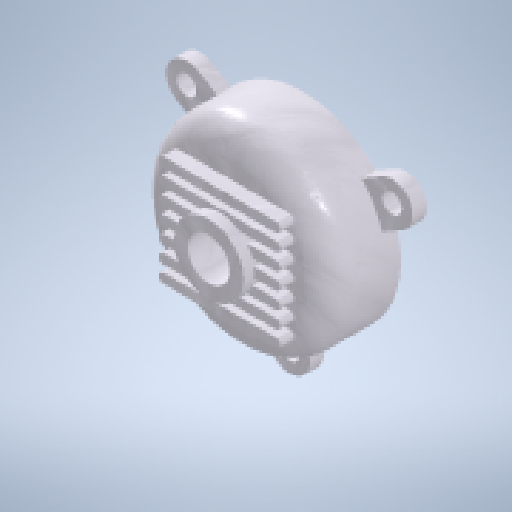
# Autodesk Inventor part: Disco do Motor Industrial
Saved by Autodesk Inventor 2023.2 (Build 272271000, 271)
## iProperties
Created: 2022-07-19
Part Number: Disco do Motor Industrial
Material: Aluminum 6061, Welded
Document SubType Name: Modeling
Designer: coqui
Density: 2.7 g/cm^3
Appearance: Weld - Aluminum
Mass: 46.1489 g
Surface Area: 212.112 cm^2
Volume: 17.0922 cm^3
Author: coqui
Autodesk Inventor part; units mm, degrees
ref_plane "YZ Plane" through (0, 0, 0) normal (1, 0, 0) x (0, 1, 0)
ref_plane "XZ Plane" through (0, 0, 0) normal (0, 1, 0) x (-1, 0, 0)
ref_plane "XY Plane" through (0, 0, 0) normal (0, 0, 1) x (1, 0, 0)
sketch "Sketch1" plane through (0, 0, 0) normal (0, 0, 1) x (1, 0, 0)
  circle A0 centre (0, 0) radius 35
  dimension "d0" = 70
  constraints: 1 centre point, 1 coincident
  measures "d0" diameter of A0
extrude "Extrusion1" add sketch "Sketch1" along normal blind 25
fillet "Fillet1" radius 10 1 edges at (-35, 0, 25)
shell "Shell1" thickness 1 removed faces 1 at (-1.9985, 11.019, 0)
sketch "Sketch2" plane through (0, 0, 0) normal (0, 0, -1) x (-1, 0, 0)
  arc A0 (-7.5, -42.5) -> (7.5, -42.5) centre (0, -42.5) ccw
  circle A1 centre (0, -42.5) radius 3.5
  line L0 (7.5, -42.5) -> (7.5, -33.6234)
  line L1 (-7.5, -42.5) -> (-7.5, -33.7627)
  arc A2 (-7.5, -33.7627) -> (7.5, -33.7627) centre (0, -11.6498) ccw
  point P0 (0, 0)
  dimension "d5" = 15
  dimension "d6" = 7
  dimension "d7" = 42.5
  constraints: 4 end point, 4 point on circle, 3 centre point, 1 coincident, 1 parallel, 1 point on line, 1 tangent, 1 vertical
  measures "d5" diameter of A0
  measures "d6" diameter of A1
  measures "d7" distance of A0.centre point (0, 0)
extrude "Extrusion2" add sketch "Sketch2" against normal blind 5
pattern_circular "Circular Pattern1" count 3 over 360 about axis through (0, 0, 15) along (0, 0, 1) of "Extrusion2"
sketch "Sketch3" plane through (0, 0, 25) normal (0, 0, 1) x (1, 0, 0)
  line L0 (20, 18) -> (-20, 18) construction
  line L1 (20, 19.75) -> (-20, 19.75)
  line L2 (-20, 16.25) -> (20, 16.25)
  arc A0 (20, 16.25) -> (20, 19.75) centre (20, 18) ccw
  arc A1 (-20, 19.75) -> (-20, 16.25) centre (-20, 18) ccw
  line L3 (0, 42.0299) -> (0, -57.656) construction
  line L4 (20, 12) -> (-20, 12) construction
  line L5 (20, 13.75) -> (-20, 13.75)
  line L6 (-20, 10.25) -> (20, 10.25)
  arc A2 (20, 10.25) -> (20, 13.75) centre (20, 12) ccw
  arc A3 (-20, 13.75) -> (-20, 10.25) centre (-20, 12) ccw
  line L7 (20, 6) -> (-20, 6) construction
  line L8 (20, 7.75) -> (-20, 7.75)
  line L9 (-20, 4.25) -> (20, 4.25)
  arc A4 (20, 4.25) -> (20, 7.75) centre (20, 6) ccw
  arc A5 (-20, 7.75) -> (-20, 4.25) centre (-20, 6) ccw
  line L10 (20, 0) -> (-20, 0) construction
  line L11 (20, 1.75) -> (-20, 1.75)
  line L12 (-20, -1.75) -> (20, -1.75)
  arc A6 (20, -1.75) -> (20, 1.75) centre (20, 0) ccw
  arc A7 (-20, 1.75) -> (-20, -1.75) centre (-20, 0) ccw
  line L13 (20, -6) -> (-20, -6) construction
  line L14 (20, -4.25) -> (-20, -4.25)
  line L15 (-20, -7.75) -> (20, -7.75)
  arc A8 (20, -7.75) -> (20, -4.25) centre (20, -6) ccw
  arc A9 (-20, -4.25) -> (-20, -7.75) centre (-20, -6) ccw
  line L16 (20, -12) -> (-20, -12) construction
  line L17 (20, -10.25) -> (-20, -10.25)
  line L18 (-20, -13.75) -> (20, -13.75)
  arc A10 (20, -13.75) -> (20, -10.25) centre (20, -12) ccw
  arc A11 (-20, -10.25) -> (-20, -13.75) centre (-20, -12) ccw
  line L19 (20, -18) -> (-20, -18) construction
  line L20 (20, -16.25) -> (-20, -16.25)
  line L21 (-20, -19.75) -> (20, -19.75)
  arc A12 (20, -19.75) -> (20, -16.25) centre (20, -18) ccw
  arc A13 (-20, -16.25) -> (-20, -19.75) centre (-20, -18) ccw
  point P0 (0, 0)
  point P1 (0, 18)
  point P2 (0, 12)
  point P3 (0, 6)
  point P4 (0, 0)
  point P5 (0, -6)
  point P6 (0, -12)
  point P7 (0, -18)
  dimension "d13" = 40
  dimension "d14" = 1.75
  dimension "d17" = 18
  dimension "d18" = 20
  dimension "d21" = 6
  constraints: 58 end point, 28 point on circle, 14 centre point, 4 tangent, 2 vertical, 1 horizontal, 1 midpoint, 1 parallel, 72 other
  measures "d13" distance of L2.start L2.end
  measures "d14" radius of A1
  measures "d17" distance of point (0, 0) point (0, 18)
  measures "d18" horizontal distance of point (0, 0) L2.start
  measures "d21" distance of L1.start L5.start
extrude "Extrusion3" add sketch "Sketch3" along normal blind 5
sketch "Sketch4" plane through (0, 0, 25) normal (0, 0, 1) x (1, 0, 0)
  circle A0 centre (0, 0) radius 12.5
  dimension "d28" = 25
  constraints: 1 centre point, 1 coincident
  measures "d28" diameter of A0
extrude "Extrusion4" add sketch "Sketch4" along normal blind 9
sketch "Sketch5" plane through (0, 0, 34) normal (0, 0, 1) x (1, 0, 0)
  circle A0 centre (0, 0) radius 7.5
  dimension "d31" = 15
  constraints: 1 centre point, 1 coincident
  measures "d31" diameter of A0
extrude "Extrusion5" cut sketch "Sketch5" against normal blind 15
body "Solid1"
